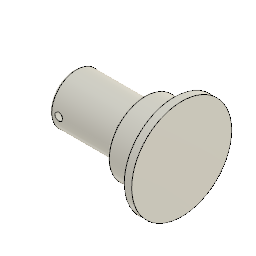
Knee Axis (Autodesk Fusion 360 design; units mm, degrees)
Autodesk Fusion 360 part; units mm, degrees
sketch "Sketch1" plane through (0, 0, 0) normal (0, 0, 1) x (1, 0, 0)
  line L0 (0, 0) -> (3, 0)
  line L1 (3, 0) -> (3, 20)
  line L2 (3, 20) -> (0, 20)
  line L3 (0, 20) -> (0, 14.5)
  line L4 (0, 0) -> (-17.5, 0)
  line L5 (-17.5, 10) -> (-17.5, 14.5)
  line L6 (-17.5, 14.5) -> (0, 14.5)
  line L7 (-17.5, 0) -> (-65, 0)
  line L8 (-65, 0) -> (-65, 10)
  line L9 (-65, 10) -> (-17.5, 10)
  dimension "d1" = 3
  dimension "d2" = 20
  dimension "d3" = 14.5
  dimension "d4" = 17.5
  dimension "d5" = 10
  dimension "d6" = 47.5
  constraint horizontal L0
  constraint vertical L1
  constraint horizontal L2
  constraint vertical L3
  constraint coincident L0.start L4.start
  constraint horizontal L4
  constraint vertical L5
  constraint horizontal L6
  constraint horizontal L7
  constraint vertical L8
  constraint horizontal L9
  measures "d1" distance of L1.end L2.end
  measures "d2" distance of L0.end L1.end
  measures "d3" distance of L4 L6
  measures "d4" distance of L5.end L3.end
  measures "d5" distance of L7 L9
  measures "d6" distance of L8.end L5.start
revolve "Revolve1" add sketch "Sketch1" angle 360 about axis through (-17.5, 0, 0) along (-1, 0, 0) makes body 1
fillet "Fillet1" radius 1 2 edges at (-65, -3.6162, 9.3233) (-17.5, -5.2434, 13.5187) on bodies 1
ref_plane "WorkPlane1" through (0, 0, 0) normal (-1, 0, 0) x (0, 0, 1)
split "Split1" by plane through (0, 0, 0) normal (-1, 0, 0) bodies 1 makes body 2 at (-48.5, 9.9876, 0.4985)
extrude "Extrude1" cut 1 faces at (0, -4.2082, 1.2981) along direction (-1, 0, 0) blind 5.35 on bodies 2 bodies 2
move_body "Move1" bodies 1 to x (1, 0, 0) y (0, 1, 0) z (0, 0, 1) at (-5.35, 0, 0)
delete_face "DeleteFace1" 1 faces at (-64.3271, -0.2479, -9.9419) on bodies 2
extrude "Extrude2" cut 1 faces at (-65, -2.7541, -1.0148) along direction (1, 0, 0) blind 4.65 on bodies 2 bodies 2
extrude "Extrude3" add 1 faces at (-2.35, 3.8604, 3.2472) along direction (1, 0, 0) blind 0.35 on bodies 1 bodies 1
extrude "Extrude4" cut 1 faces at (-5.35, 4.7423, 7.1112) along direction (1, 0, 0) blind 0.35 on bodies 1 bodies 1
extrude "Extrude5" cut 1 faces at (-60.35, -2.7541, -1.0148) along direction (1, 0, 0) blind 15.35 on bodies 2 bodies 2
fillet "Fillet3" radius 1 1 edges at (-45, -9.3233, -3.6162) on bodies 2
extrude "Extrude6" add 1 faces at (-5.35, -4.2082, 1.2981) along direction (1, 0, 0) blind 3 on bodies 2 bodies 2 1
hole "Hole1" at (-41.2, -10, 0) direction (0, 1, 0) diameter 3 end through all bodies 2
equation "d6 = 50 mm - 2.5 mm"
